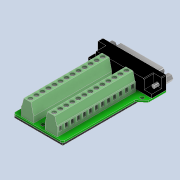
# Autodesk Inventor part: 25Pin D SUB Male Connector
Saved by Autodesk Inventor 2022 (Build 260153000, 153)
## iProperties
Created: 2021-12-24
Part Number: 25Pin D SUB Male Connector
Material: Generic
Document SubType Name: Modeling
Designer: Coy
Density: 1 g/cm^3
Appearance: Anodized - Black
Author: Coy
Autodesk Inventor part; units mm, degrees
ref_plane "YZ Plane" through (0, 0, 0) normal (1, 0, 0) x (0, 1, 0)
ref_plane "XZ Plane" through (0, 0, 0) normal (0, 1, 0) x (-1, 0, 0)
sketch "Sketch1" plane through (0, 0, 0) normal (0, 1, 0) x (-1, 0, 0)
  line L0 (0, 0) -> (53, 0)
  line L1 (53, 0) -> (53, -80)
  line L2 (53, -80) -> (0, -80)
  line L3 (0, -80) -> (0, 0)
  line L4 (47, 0) -> (47, -60)
  line L5 (47, -60) -> (53, -65)
  line L6 (26.5, -80) -> (26.5, 0) construction
  line L7 (6, 0) -> (6, -60)
  line L8 (6, -60) -> (0, -65)
  dimension "d0" = 53
  dimension "d1" = 80
  dimension "d2" = 60
  dimension "d3" = 6
  dimension "d4" = 15
  constraints: 18 end point, 3 symmetric about line, 2 midpoint, 2 parallel, 2 point on line, 1 horizontal, 1 perpendicular, 1 vertical
  measures "d0" distance of L1.end L2.end
  measures "d1" distance of L0.end L1.end
  measures "d2" distance of L4.start L4.end
  measures "d3" distance between parallel lines of L1 L4
  measures "d4" distance of L1.end L5.end
extrude "Extrusion1" add sketch "Sketch1" along normal blind 1.5 contours L0 L4 L5 L1 L2 L3 L8 L7
sketch "Sketch2" plane through (0, 0, 0) normal (0, -1, 0) x (1, 0, 0)
  line L0 (-46.5, -0.5) -> (-6.5, -0.5)
  line L1 (-6.5, -0.5) -> (-6.5, -79.5)
  line L2 (-6.5, -79.5) -> (-46.5, -79.5)
  line L3 (-46.5, -79.5) -> (-46.5, -0.5)
  line L4 (-47, 0) -> (-6, 0) projected
  line L5 (-47, -60) -> (-47, 0) projected
  line L6 (-6, 0) -> (-6, -60) projected
  line L7 (0, -80) -> (-53, -80) projected
  point P0 (0, 0)
  dimension "d7" = 0.5
  dimension "d8" = 0.5
  dimension "d9" = 0.5
  dimension "d10" = 0.5
  constraints: 8 end point, 2 parallel, 1 horizontal, 1 perpendicular
  measures "d7" distance between parallel lines of L4 L0
  measures "d8" distance between parallel lines of L5 L3
  measures "d9" distance between parallel lines of L6 L1
  measures "d10" distance between parallel lines of L7 L2
extrude "Extrusion2" add sketch "Sketch2" along normal blind 2
sketch "Sketch3" plane through (0, 1.5, 0) normal (0, 1, 0) x (1, 0, 0)
  line L0 (-4.625, -3.6868) -> (-4.625, 83.4711) construction
  line L1 (-48.625, -3.6868) -> (-48.625, 83.4711) construction
  line L2 (0, 65) -> (0, 80) construction
  line L3 (15.3473, 64.5) -> (-90.3777, 64.5) construction
  line L4 (0, 80) -> (-53, 80) construction
  line L5 (0, 80) -> (-53, 80) construction
  line L6 (-26.5, 80) -> (-26.5, 0) construction
  line L7 (-47, 0) -> (-6, 0) construction
  line L8 (-6, 0) -> (-6, 60) construction
  line L9 (-6, 4) -> (-47, 4) construction
  line L10 (-47, 60) -> (-47, 0) construction
  circle A0 centre (-26.5, 4) radius 1.625
  circle A1 centre (-4.625, 64.5) radius 1.625
  circle A2 centre (-48.625, 64.5) radius 1.625
  point P0 (0, 0)
  dimension "d13" = 44
  dimension "d14" = 4.625
  dimension "d15" = 15.5
  dimension "d16" = 4
  dimension "d17" = 3.25
  dimension "d18" = 3.25
  dimension "d19" = 3.25
  constraints: 10 end point, 6 point on line, 3 centre point, 3 midpoint, 2 horizontal, 2 vertical
  measures "d13" distance between parallel lines of L1 L0
  measures "d14" distance between parallel lines of L2 L0
  measures "d15" distance between parallel lines of L4 L3
  measures "d16" distance between parallel lines of L7 L9
  measures "d17" diameter of A0
  measures "d18" diameter of A1
  measures "d19" diameter of A2
extrude "Extrusion3" cut sketch "Sketch3" against normal up to surface (1.5 mm away)
sketch "Sketch4" plane through (0, 1.5, 0) normal (0, 1, 0) x (1, 0, 0)
  line L0 (-53, 80) -> (-53, 65) projected
  line L1 (0, 65) -> (0, 80) projected
  line L2 (-53, 80) -> (0, 80)
  line L3 (0, 80) -> (0, 68)
  line L4 (0, 68) -> (-53, 68)
  line L5 (-53, 68) -> (-53, 80)
  point P0 (0, 0)
  dimension "d22" = 12
  constraints: 8 end point, 2 parallel, 1 horizontal, 1 perpendicular, 1 point on line
  measures "d22" distance of L2.end L3.end
extrude "Extrusion4" add sketch "Sketch4" along normal blind 3
sketch "Sketch5" plane through (0, 4.5, 0) normal (0, 1, 0) x (1, 0, 0)
  line L0 (-53, 80) -> (-53, 68) projected
  line L1 (-53, 68) -> (0, 68) projected
  line L2 (0, 68) -> (0, 80) projected
  line L3 (0, 80) -> (-53, 80) projected
  line L4 (-53, 80) -> (-53, 65) projected
  line L5 (-53, 76) -> (0.4812, 76)
  line L6 (-46.5, 76) -> (-46.5, 68)
  line L7 (0, 68) -> (-53, 68) projected
  line L8 (-6.5, 76) -> (-6.5, 68)
  point P0 (0, 0)
  point P1 (0, 76)
  dimension "d25" = 4
  dimension "d26" = 6.5
  dimension "d27" = 6.5
  constraints: 6 end point, 5 point on line, 2 perpendicular, 1 horizontal
  measures "d25" distance between parallel lines of L3 L5
  measures "d26" distance between parallel lines of L0 L6
  measures "d27" distance between parallel lines of L2 L8
extrude "Extrusion5" add sketch "Sketch5" along normal blind 8 contours L3 L2 L5 L0 | L5 L8 L1 L6
sketch "Sketch6" plane through (0, 0, -80) normal (0, 0, -1) x (-1, 0, 0)
  line L0 (7.25, 10.25) -> (45.75, 10.25)
  line L1 (43.75, 2.25) -> (9.25, 2.25)
  line L2 (43.75, 10.25) -> (43.75, 2.25) construction
  line L3 (9.25, 10.25) -> (9.25, 2.25) construction
  line L4 (7.25, 10.25) -> (9.25, 2.25)
  line L5 (43.75, 2.25) -> (45.75, 10.25)
  line L6 (46.5, 12.5) -> (6.5, 12.5) construction
  line L7 (26.5, 12.5) -> (26.5, -2) construction
  line L8 (46.5, -2) -> (6.5, -2) construction
  line L9 (0, 0) -> (0, 12.5) construction
  line L10 (0, 6.25) -> (53, 6.25) construction
  line L11 (53, 0) -> (53, 12.5) construction
  line L12 (4.527, 8.575) -> (5.8694, 6.25)
  line L13 (5.8694, 6.25) -> (4.527, 3.925)
  line L14 (4.527, 3.925) -> (1.8423, 3.925)
  line L15 (1.8423, 3.925) -> (0.5, 6.25)
  line L16 (0.5, 6.25) -> (1.8423, 8.575)
  line L17 (1.8423, 8.575) -> (4.527, 8.575)
  line L18 (51.1577, 8.575) -> (52.5, 6.25)
  line L19 (52.5, 6.25) -> (51.1577, 3.925)
  line L20 (51.1577, 3.925) -> (48.473, 3.925)
  line L21 (48.473, 3.925) -> (47.1306, 6.25)
  line L22 (47.1306, 6.25) -> (48.473, 8.575)
  line L23 (48.473, 8.575) -> (51.1577, 8.575)
  point P0 (3.1847, 6.25)
  point P1 (49.8153, 6.25)
  point P2 (49.8153, 8.575)
  dimension "d34" = 38.5
  dimension "d35" = 8
  dimension "d36" = 104.036
  dimension "d37" = 104.036
  dimension "d38" = 19.25
  dimension "d39" = 4
  dimension "d40" = 4.65
  dimension "d41" = 4.65
  dimension "d42" = 0.5
  dimension "d43" = 0.5
  constraints: 40 end point, 5 midpoint, 5 point on line, 2 horizontal, 2 perpendicular, 1 parallel, 26 other
  measures "d34" distance of L0.start L0.end
  measures "d35" distance between parallel lines of L1 L0
  measures "d36" angle of L1 L4
  measures "d37" angle of L1 L5
  measures "d38" distance from line of L7 L0.end
  measures "d39" distance between parallel lines of L10 L0
  measures "d40" distance between parallel lines of L14 L17
  measures "d41" distance between parallel lines of L20 L23
  measures "d42" distance from line of L11 L18.end
  measures "d43" distance of L10.start L15.end
extrude "Extrusion6" add sketch "Sketch6" along normal blind 6.25
sketch "Sketch7" plane through (0, 0, -86.25) normal (0, 0, -1) x (-1, 0, 0)
  line L0 (1.8423, 8.575) -> (0.5, 6.25) projected
  line L1 (0.5, 6.25) -> (1.8423, 3.925) projected
  line L2 (1.8423, 3.925) -> (4.527, 3.925) projected
  line L3 (4.527, 3.925) -> (5.8694, 6.25) projected
  line L4 (5.8694, 6.25) -> (4.527, 8.575) projected
  line L5 (4.527, 8.575) -> (1.8423, 8.575) projected
  line L6 (48.473, 8.575) -> (47.1306, 6.25) projected
  line L7 (47.1306, 6.25) -> (48.473, 3.925) projected
  line L8 (48.473, 3.925) -> (51.1577, 3.925) projected
  line L9 (51.1577, 3.925) -> (52.5, 6.25) projected
  line L10 (52.5, 6.25) -> (51.1577, 8.575) projected
  line L11 (51.1577, 8.575) -> (48.473, 8.575) projected
  circle A0 centre (3.1847, 6.25) radius 1.25
  circle A1 centre (49.8153, 6.25) radius 1.25
  line L12 (45.75, 10.25) -> (7.25, 10.25) projected
  line L13 (7.25, 10.25) -> (9.25, 2.25) projected
  line L14 (9.25, 2.25) -> (43.75, 2.25) projected
  line L15 (43.75, 2.25) -> (45.75, 10.25) projected
  line L16 (7.8904, 9.75) -> (45.1096, 9.75)
  line L17 (45.1096, 9.75) -> (43.3596, 2.75)
  line L18 (43.3596, 2.75) -> (9.6404, 2.75)
  line L19 (9.6404, 2.75) -> (7.8904, 9.75)
  line L20 (9.6404, 7.25) -> (43.3596, 7.25) construction
  line L21 (9.6404, 5.25) -> (43.3596, 5.25) construction
  circle A2 centre (9.6404, 7.25) radius 0.5
  circle A3 centre (12.4404, 7.25) radius 0.5
  circle A4 centre (15.2404, 7.25) radius 0.5
  circle A5 centre (18.0404, 7.25) radius 0.5
  circle A6 centre (20.8404, 7.25) radius 0.5
  circle A7 centre (23.6404, 7.25) radius 0.5
  circle A8 centre (26.4404, 7.25) radius 0.5
  circle A9 centre (29.2404, 7.25) radius 0.5
  circle A10 centre (32.0404, 7.25) radius 0.5
  circle A11 centre (34.8404, 7.25) radius 0.5
  circle A12 centre (37.6404, 7.25) radius 0.5
  circle A13 centre (40.4404, 7.25) radius 0.5
  circle A14 centre (43.2404, 7.25) radius 0.5
  circle A15 centre (11.0404, 5.25) radius 0.5
  circle A16 centre (13.8404, 5.25) radius 0.5
  circle A17 centre (16.6404, 5.25) radius 0.5
  circle A18 centre (19.4404, 5.25) radius 0.5
  circle A19 centre (22.2404, 5.25) radius 0.5
  circle A20 centre (25.0404, 5.25) radius 0.5
  circle A21 centre (27.8404, 5.25) radius 0.5
  circle A22 centre (30.6404, 5.25) radius 0.5
  circle A23 centre (33.4404, 5.25) radius 0.5
  circle A24 centre (36.2404, 5.25) radius 0.5
  circle A25 centre (39.0404, 5.25) radius 0.5
  circle A26 centre (41.8404, 5.25) radius 0.5
  point P0 (0, 0)
  dimension "d46" = 2.5
  dimension "d47" = 2.5
  dimension "d48" = 0.5
  dimension "d49" = 3
  dimension "d50" = 3
  dimension "d51" = 1
  dimension "d54" = 2.8
  dimension "d59" = 1
  dimension "d60" = 1.4
  dimension "d63" = 2.8
  constraints: 27 centre point, 12 end point, 3 horizontal, 1 coincident, 1 parallel, 1 point on line, 49 other
  measures "d46" diameter of A0
  measures "d47" diameter of A1
  measures "d48" distance between parallel lines of L12 L16
  measures "d49" distance between parallel lines of L12 L20
  measures "d50" distance between parallel lines of L14 L21
  measures "d51" diameter of A2
  measures "d54" distance of A2.centre A3.centre
  measures "d59" diameter of A15
  measures "d60" horizontal distance of L20.start A15.centre
  measures "d63" distance of A15.centre A16.centre
extrude "Extrusion7" cut sketch "Sketch7" against normal up to surface (6.25 mm away) contours A0 | A1 | L16 L17 L18 L19
sketch "Sketch8" plane through (-6.5, 4.5, -76) normal (0, 0, 1) x (1, 0, 0)
  circle A0 centre (-43.3153, 1.75) radius 1.25 projected
  circle A1 centre (3.3153, 1.75) radius 1.25 projected
  circle A2 centre (-43.3153, 1.75) radius 1.25 projected
  circle A3 centre (-43.3153, 1.75) radius 1.5
  circle A4 centre (3.3153, 1.75) radius 1.25 projected
  circle A5 centre (3.3153, 1.75) radius 1.5
  point P0 (6.5, -4.5)
  dimension "d70" = 3
  dimension "d71" = 3
  constraints: 2 centre point, 2 coincident
  measures "d70" diameter of A3
  measures "d71" diameter of A5
extrude "Extrusion8" add sketch "Sketch8" along normal blind 3.5 contours A0 | A1 | A3 | A5
ref_plane "Work Plane1" through (-47, 0, -1) normal (0, 0, 1) x (1, 0, 0)
sketch "Sketch9" plane through (-47, 0, -1) normal (0, 0, 1) x (1, 0, 0)
  line L0 (47, 0) -> (-6, 0) construction
  line L1 (20.5, 0) -> (20.5, 19.9001) construction
  line L2 (47, 1.5) -> (-6, 1.5) construction
  line L3 (5.5, 1.5) -> (5.5, 9.25)
  line L4 (5.5, 9.25) -> (6, 9.25)
  line L5 (6, 9.25) -> (7.625, 15.5)
  line L6 (7.625, 15.5) -> (13.625, 15.5)
  line L7 (13.625, 15.5) -> (15.75, 6.5)
  line L8 (15.75, 6.5) -> (15.75, 1.5)
  line L9 (0, 1.5) -> (41, 1.5) projected
  line L10 (5.5, 2.0746) -> (15.75, 2.0746) construction
  line L11 (10.625, 2.0746) -> (10.625, 15.5) construction
  line L12 (0, 0) -> (0, 1.5) construction
  line L13 (35.5, 1.5) -> (35.5, 9.25)
  line L14 (35.5, 9.25) -> (35, 9.25)
  line L15 (35, 9.25) -> (33.375, 15.5)
  line L16 (33.375, 15.5) -> (27.375, 15.5)
  line L17 (27.375, 15.5) -> (25.25, 6.5)
  line L18 (25.25, 6.5) -> (25.25, 1.5)
  line L19 (35.5, 2.0746) -> (25.25, 2.0746) construction
  line L20 (30.375, 2.0746) -> (30.375, 15.5) construction
  dimension "d75" = 14
  dimension "d76" = 7.75
  dimension "d77" = 0.5
  dimension "d78" = 5
  dimension "d79" = 6
  dimension "d80" = 10.25
  dimension "d81" = 5.5
  constraints: 34 end point, 11 symmetric about line, 6 point on line, 3 midpoint, 3 perpendicular, 2 parallel, 2 vertical
  measures "d75" distance between parallel lines of L2 L6
  measures "d76" distance of L3.start L3.end
  measures "d77" distance of L3.end L4.end
  measures "d78" distance of L7.end L8.end
  measures "d79" distance of L5.end L6.end
  measures "d80" distance of L8.end L3.start
  measures "d81" distance between parallel lines of L12 L3
extrude "Extrusion9" add sketch "Sketch9" against normal blind 65
sketch "Sketch10" plane through (-19.625, 15.5, -1) normal (0, 1, 0) x (1, 0, 0)
  line L0 (-21.875, 65) -> (-11.625, 65) construction
  line L1 (-16.75, 65) -> (-16.75, 0) construction
  line L2 (-11.625, 0) -> (-21.875, 0) construction
  line L3 (-27.375, -1) -> (13.625, -1) construction
  line L4 (-6.3154, 85.25) -> (-7.3154, 85.25) construction
  line L5 (-6.875, -1) -> (-6.875, 85.2511) construction
  circle A0 centre (-16.75, 2.5) radius 1.875
  circle A1 centre (-16.75, 7.5) radius 1.875
  circle A2 centre (-16.75, 12.5) radius 1.875
  circle A3 centre (-16.75, 17.5) radius 1.875
  circle A4 centre (-16.75, 22.5) radius 1.875
  circle A5 centre (-16.75, 27.5) radius 1.875
  circle A6 centre (-16.75, 32.5) radius 1.875
  circle A7 centre (-16.75, 37.5) radius 1.875
  circle A8 centre (-16.75, 42.5) radius 1.875
  circle A9 centre (-16.75, 47.5) radius 1.875
  circle A10 centre (-16.75, 52.5) radius 1.875
  circle A11 centre (-16.75, 57.5) radius 1.875
  circle A12 centre (-16.75, 62.5) radius 1.875
  line L6 (3, 65) -> (3, 0) construction
  circle A13 centre (3, 2.5) radius 1.875
  circle A14 centre (3, 7.5) radius 1.875
  circle A15 centre (3, 12.5) radius 1.875
  circle A16 centre (3, 17.5) radius 1.875
  circle A17 centre (3, 22.5) radius 1.875
  circle A18 centre (3, 27.5) radius 1.875
  circle A19 centre (3, 32.5) radius 1.875
  circle A20 centre (3, 37.5) radius 1.875
  circle A21 centre (3, 42.5) radius 1.875
  circle A22 centre (3, 47.5) radius 1.875
  circle A23 centre (3, 52.5) radius 1.875
  circle A24 centre (3, 57.5) radius 1.875
  circle A25 centre (3, 62.5) radius 1.875
  point P0 (19.625, -1)
  point P1 (-2.125, 65)
  point P2 (-2.125, 0)
  dimension "d84" = 3.75
  dimension "d85" = 2.5
  dimension "d88" = 5
  constraints: 26 centre point, 17 symmetric about line, 6 end point, 3 midpoint, 2 point on line, 1 perpendicular, 1 vertical, 37 other
  measures "d84" diameter of A0
  measures "d85" distance from line of L2 A0.centre
  measures "d88" distance of A0.centre A1.centre
extrude "Extrusion10" cut sketch "Sketch10" against normal blind 1.5
sketch "Sketch11" plane through (-11.5, 1.5, -1) normal (1, 0, 0) x (0, 0, -1)
  line L0 (1.25, 6.75) -> (3.75, 6.75)
  line L1 (3.75, 6.75) -> (3.75, 2.75)
  line L2 (3.75, 2.75) -> (1.25, 2.75)
  line L3 (1.25, 2.75) -> (1.25, 6.75)
  line L4 (0.625, 14) -> (4.375, 14) construction
  line L5 (2.5, 14) -> (2.5, 0) construction
  line L6 (59, 0) -> (-1, 0) construction
  line L7 (0, 7.75) -> (65, 7.75) construction
  line L8 (6.25, 6.75) -> (8.75, 6.75)
  line L9 (8.75, 6.75) -> (8.75, 2.75)
  line L10 (8.75, 2.75) -> (6.25, 2.75)
  line L11 (6.25, 2.75) -> (6.25, 6.75)
  line L12 (7.5, 14) -> (7.5, 0) construction
  line L13 (11.25, 6.75) -> (13.75, 6.75)
  line L14 (13.75, 6.75) -> (13.75, 2.75)
  line L15 (13.75, 2.75) -> (11.25, 2.75)
  line L16 (11.25, 2.75) -> (11.25, 6.75)
  line L17 (12.5, 14) -> (12.5, 0) construction
  line L18 (16.25, 6.75) -> (18.75, 6.75)
  line L19 (18.75, 6.75) -> (18.75, 2.75)
  line L20 (18.75, 2.75) -> (16.25, 2.75)
  line L21 (16.25, 2.75) -> (16.25, 6.75)
  line L22 (17.5, 14) -> (17.5, 0) construction
  line L23 (21.25, 6.75) -> (23.75, 6.75)
  line L24 (23.75, 6.75) -> (23.75, 2.75)
  line L25 (23.75, 2.75) -> (21.25, 2.75)
  line L26 (21.25, 2.75) -> (21.25, 6.75)
  line L27 (22.5, 14) -> (22.5, 0) construction
  line L28 (26.25, 6.75) -> (28.75, 6.75)
  line L29 (28.75, 6.75) -> (28.75, 2.75)
  line L30 (28.75, 2.75) -> (26.25, 2.75)
  line L31 (26.25, 2.75) -> (26.25, 6.75)
  line L32 (27.5, 14) -> (27.5, 0) construction
  line L33 (31.25, 6.75) -> (33.75, 6.75)
  line L34 (33.75, 6.75) -> (33.75, 2.75)
  line L35 (33.75, 2.75) -> (31.25, 2.75)
  line L36 (31.25, 2.75) -> (31.25, 6.75)
  line L37 (32.5, 14) -> (32.5, 0) construction
  line L38 (36.25, 6.75) -> (38.75, 6.75)
  line L39 (38.75, 6.75) -> (38.75, 2.75)
  line L40 (38.75, 2.75) -> (36.25, 2.75)
  line L41 (36.25, 2.75) -> (36.25, 6.75)
  line L42 (37.5, 14) -> (37.5, 0) construction
  line L43 (41.25, 6.75) -> (43.75, 6.75)
  line L44 (43.75, 6.75) -> (43.75, 2.75)
  line L45 (43.75, 2.75) -> (41.25, 2.75)
  line L46 (41.25, 2.75) -> (41.25, 6.75)
  line L47 (42.5, 14) -> (42.5, 0) construction
  line L48 (46.25, 6.75) -> (48.75, 6.75)
  line L49 (48.75, 6.75) -> (48.75, 2.75)
  line L50 (48.75, 2.75) -> (46.25, 2.75)
  line L51 (46.25, 2.75) -> (46.25, 6.75)
  line L52 (47.5, 14) -> (47.5, 0) construction
  line L53 (51.25, 6.75) -> (53.75, 6.75)
  line L54 (53.75, 6.75) -> (53.75, 2.75)
  line L55 (53.75, 2.75) -> (51.25, 2.75)
  line L56 (51.25, 2.75) -> (51.25, 6.75)
  line L57 (52.5, 14) -> (52.5, 0) construction
  line L58 (56.25, 6.75) -> (58.75, 6.75)
  line L59 (58.75, 6.75) -> (58.75, 2.75)
  line L60 (58.75, 2.75) -> (56.25, 2.75)
  line L61 (56.25, 2.75) -> (56.25, 6.75)
  line L62 (57.5, 14) -> (57.5, 0) construction
  line L63 (61.25, 6.75) -> (63.75, 6.75)
  line L64 (63.75, 6.75) -> (63.75, 2.75)
  line L65 (63.75, 2.75) -> (61.25, 2.75)
  line L66 (61.25, 2.75) -> (61.25, 6.75)
  line L67 (62.5, 14) -> (62.5, 0) construction
  point P0 (-1, -1.5)
  dimension "d95" = 2.5
  dimension "d96" = 4
  dimension "d97" = 1.25
  dimension "d98" = 1
  dimension "d101" = 5
  constraints: 130 end point, 2 horizontal, 2 parallel, 1 midpoint, 1 perpendicular, 1 point on line, 1 vertical, 132 other
  measures "d95" distance of L1.end L2.end
  measures "d96" distance of L0.end L1.end
  measures "d97" distance between parallel lines of L5 L1
  measures "d98" distance between parallel lines of L7 L0
  measures "d101" distance of L0.start L8.start
extrude "Extrusion11" cut sketch "Sketch11" against normal blind 2
sketch "Sketch12" plane through (-41.5, 1.5, -1) normal (-1, 0, 0) x (0, 0, 1)
  line L0 (-13.75, 6.75) -> (-13.75, 2.75) projected
  line L1 (-13.75, 2.75) -> (-11.25, 2.75) projected
  line L2 (-11.25, 2.75) -> (-11.25, 6.75) projected
  line L3 (-11.25, 6.75) -> (-13.75, 6.75) projected
  line L4 (-33.75, 6.75) -> (-33.75, 2.75) projected
  line L5 (-33.75, 2.75) -> (-31.25, 2.75) projected
  line L6 (-31.25, 2.75) -> (-31.25, 6.75) projected
  line L7 (-31.25, 6.75) -> (-33.75, 6.75) projected
  line L8 (-53.75, 6.75) -> (-53.75, 2.75) projected
  line L9 (-53.75, 2.75) -> (-51.25, 2.75) projected
  line L10 (-51.25, 2.75) -> (-51.25, 6.75) projected
  line L11 (-51.25, 6.75) -> (-53.75, 6.75) projected
  line L12 (-58.75, 6.75) -> (-58.75, 2.75) projected
  line L13 (-58.75, 2.75) -> (-56.25, 2.75) projected
  line L14 (-56.25, 2.75) -> (-56.25, 6.75) projected
  line L15 (-56.25, 6.75) -> (-58.75, 6.75) projected
  line L16 (-38.75, 6.75) -> (-38.75, 2.75) projected
  line L17 (-38.75, 2.75) -> (-36.25, 2.75) projected
  line L18 (-36.25, 2.75) -> (-36.25, 6.75) projected
  line L19 (-36.25, 6.75) -> (-38.75, 6.75) projected
  line L20 (-18.75, 6.75) -> (-18.75, 2.75) projected
  line L21 (-18.75, 2.75) -> (-16.25, 2.75) projected
  line L22 (-16.25, 2.75) -> (-16.25, 6.75) projected
  line L23 (-16.25, 6.75) -> (-18.75, 6.75) projected
  line L24 (-8.75, 6.75) -> (-8.75, 2.75) projected
  line L25 (-8.75, 2.75) -> (-6.25, 2.75) projected
  line L26 (-6.25, 2.75) -> (-6.25, 6.75) projected
  line L27 (-6.25, 6.75) -> (-8.75, 6.75) projected
  line L28 (-28.75, 6.75) -> (-28.75, 2.75) projected
  line L29 (-28.75, 2.75) -> (-26.25, 2.75) projected
  line L30 (-26.25, 2.75) -> (-26.25, 6.75) projected
  line L31 (-26.25, 6.75) -> (-28.75, 6.75) projected
  line L32 (-48.75, 6.75) -> (-48.75, 2.75) projected
  line L33 (-48.75, 2.75) -> (-46.25, 2.75) projected
  line L34 (-46.25, 2.75) -> (-46.25, 6.75) projected
  line L35 (-46.25, 6.75) -> (-48.75, 6.75) projected
  line L36 (-63.75, 6.75) -> (-63.75, 2.75) projected
  line L37 (-63.75, 2.75) -> (-61.25, 2.75) projected
  line L38 (-61.25, 2.75) -> (-61.25, 6.75) projected
  line L39 (-61.25, 6.75) -> (-63.75, 6.75) projected
  line L40 (-43.75, 6.75) -> (-43.75, 2.75) projected
  line L41 (-43.75, 2.75) -> (-41.25, 2.75) projected
  line L42 (-41.25, 2.75) -> (-41.25, 6.75) projected
  line L43 (-41.25, 6.75) -> (-43.75, 6.75) projected
  line L44 (-23.75, 6.75) -> (-23.75, 2.75) projected
  line L45 (-23.75, 2.75) -> (-21.25, 2.75) projected
  line L46 (-21.25, 2.75) -> (-21.25, 6.75) projected
  line L47 (-21.25, 6.75) -> (-23.75, 6.75) projected
  line L48 (-3.75, 6.75) -> (-3.75, 2.75) projected
  line L49 (-3.75, 2.75) -> (-1.25, 2.75) projected
  line L50 (-1.25, 2.75) -> (-1.25, 6.75) projected
  line L51 (-1.25, 6.75) -> (-3.75, 6.75) projected
  line L52 (0, 0) -> (0, 7.75) projected
  line L53 (-65, 0) -> (0, 0) projected
  line L54 (-65, 7.75) -> (-65, 0) projected
  line L55 (0, 7.75) -> (-65, 7.75) projected
  point P0 (1, -1.5)
extrude "Extrusion12" cut sketch "Sketch12" against normal blind 2 contours L3 L2 L1 L0 | L7 L6 L5 L4 | L11 L10 L9 L8 | L15 L14 L13 L12 | L19 L18 L17 L16 | L23 L22 L21 L20 | L27 L26 L25 L24 | L31 L30 L29 L28 | L35 L34 L33 L32 | L39 L38 L37 L36 | L43 L42 L41 L40 | L47 L46 L45 L44 | L51 L50 L49 L48
fillet "Fillet1" radius 2 8 edges at (-45.1096, 9.75, -83.125) (-43.3596, 2.75, -83.125) (-7.8904, 9.75, -83.125) (-9.6404, 2.75, -83.125) (-7.25, 10.25, -83.125) (-9.25, 2.25, -83.125) (-45.75, 10.25, -83.125) (-43.75, 2.25, -83.125)
fillet "Fillet2" radius 0.5 4 edges at (-6.5, 12.5, -72) (0, 12.5, -78) (-46.5, 12.5, -72) (-53, 12.5, -78)
sketch "Sketch13" plane through (0, 0, -65) normal (1, 0, 0) x (0, 0, -1)
  line L0 (11, 12) -> (15, 12) projected
  line L1 (11, 4.5) -> (11, 12) projected
  line L2 (3, 4.5) -> (11, 4.5) projected
  line L3 (3, 1.5) -> (3, 4.5) projected
  line L4 (0, 1.5) -> (3, 1.5) projected
  line L5 (0, 0) -> (0, 1.5) projected
  line L6 (0, 0) -> (15, 0) projected
  line L7 (15, 0) -> (15, 12) projected
  line L8 (3, 1.5) -> (3, 4.5) projected
  line L9 (3, 1.5) -> (15, 1.5)
  line L10 (15, 0) -> (15, 12) projected
  point P0 (-65, 0)
  constraints: 2 end point, 1 horizontal, 1 point on line
extrude "Extrusion13" cut sketch "Sketch13" against normal blind 0.0001 contours L0 L7 L9 L3 L2 L1
sketch "Sketch14" plane through (0, 0, -80) normal (0, 0, -1) x (-1, 0, 0)
  line L0 (0, 12) -> (0.0001, 12) projected
  line L1 (0.0001, 12) -> (0.0001, 1.5) projected
  line L2 (0.0001, 1.5) -> (0, 1.5) projected
  line L3 (0, 0) -> (0, 1.5) projected
  line L4 (0, 0) -> (53, 0) projected
  line L5 (53, 0) -> (53, 12) projected
  arc A0 (53, 12) -> (52.5, 12.5) centre (52.5, 12) ccw projected
  line L6 (0.5, 12.5) -> (52.5, 12.5) projected
  arc A1 (0.5, 12.5) -> (0, 12) centre (0.5, 12) ccw projected
  line L7 (1.8423, 8.575) -> (4.527, 8.575) projected
  line L8 (4.527, 8.575) -> (5.8694, 6.25) projected
  line L9 (5.8694, 6.25) -> (4.527, 3.925) projected
  line L10 (4.527, 3.925) -> (1.8423, 3.925) projected
  line L11 (1.8423, 3.925) -> (0.5, 6.25) projected
  line L12 (0.5, 6.25) -> (1.8423, 8.575) projected
  line L13 (45.1287, 7.7649) -> (44.1287, 3.7649) projected
  arc A2 (42.1884, 2.25) -> (44.1287, 3.7649) centre (42.1884, 4.25) ccw projected
  line L14 (42.1884, 2.25) -> (10.8116, 2.25) projected
  arc A3 (8.8713, 3.7649) -> (10.8116, 2.25) centre (10.8116, 4.25) ccw projected
  line L15 (8.8713, 3.7649) -> (7.8713, 7.7649) projected
  arc A4 (9.8116, 10.25) -> (7.8713, 7.7649) centre (9.8116, 8.25) ccw projected
  line L16 (9.8116, 10.25) -> (43.1884, 10.25) projected
  arc A5 (45.1287, 7.7649) -> (43.1884, 10.25) centre (43.1884, 8.25) ccw projected
  line L17 (48.473, 8.575) -> (51.1577, 8.575) projected
  line L18 (51.1577, 8.575) -> (52.5, 6.25) projected
  line L19 (52.5, 6.25) -> (51.1577, 3.925) projected
  line L20 (51.1577, 3.925) -> (48.473, 3.925) projected
  line L21 (48.473, 3.925) -> (47.1306, 6.25) projected
  line L22 (47.1306, 6.25) -> (48.473, 8.575) projected
  line L23 (0, 1.5) -> (53, 1.5)
  line L24 (53, 1.5) -> (47, 1.5) projected
  constraints: 2 end point, 1 collinear, 1 point on line
extrude "Extrusion14" cut sketch "Sketch14" against normal blind 0.0001 contours A1 L6 A0 L5 L23 L1
sketch "Sketch15" plane through (-53, 0, -80) normal (-1, 0, 0) x (0, 0, 1)
  line L0 (0.0001, 1.5) -> (0.0001, 12) projected
  line L1 (4, 12) -> (0.0001, 12) projected
  line L2 (4, 4.5) -> (4, 12) projected
  line L3 (12, 4.5) -> (4, 4.5) projected
  line L4 (12, 1.5) -> (12, 4.5) projected
  line L5 (0.0001, 1.5) -> (12, 1.5) projected
  point P0 (80, 0)
extrude "Extrusion15" cut sketch "Sketch15" against normal blind 0.0001
fillet "Fillet3" radius 0.5 25 edges at (-9.1404, 7.25, -86.25) (-11.9404, 7.25, -86.25) (-13.3404, 5.25, -86.25) (-10.5404, 5.25, -86.25) (-14.7404, 7.25, -86.25) (-16.1404, 5.25, -86.25) (-17.5404, 7.25, -86.25) (-18.9404, 5.25, -86.25) (-20.3404, 7.25, -86.25) (-21.7404, 5.25, -86.25) (-23.1404, 7.25, -86.25) (-24.5404, 5.25, -86.25) (-27.3404, 5.25, -86.25) (-25.9404, 7.25, -86.25) (-28.7404, 7.25, -86.25) (-30.1404, 5.25, -86.25) (-31.5404, 7.25, -86.25) (-32.9404, 5.25, -86.25) (-34.3404, 7.25, -86.25) (-35.7404, 5.25, -86.25) (-37.1404, 7.25, -86.25) (-38.5404, 5.25, -86.25) (-39.9404, 7.25, -86.25) (-41.3404, 5.25, -86.25) (-42.7404, 7.25, -86.25)
thread "Thread1" size "M3x0.5" class "6g" standard "ANSI Metric M Profile" full length
thread "Thread2" size "M3x0.5" class "6g" standard "ANSI Metric M Profile" full length
chamfer "Chamfer1" distance 1.5 angle 45 26 edges at (-13.5, 8.25, -63.5) (-13.5, 8.25, -58.5) (-13.5, 8.25, -53.5) (-13.5, 8.25, -48.5) (-13.5, 8.25, -43.5) (-13.5, 8.25, -38.5) (-13.5, 8.25, -33.5) (-13.5, 8.25, -28.5) (-13.5, 8.25, -23.5) (-13.5, 8.25, -18.5) (-13.5, 8.25, -13.5) (-13.5, 8.25, -8.5) (-13.5, 8.25, -3.5) (-39.5, 8.25, -63.5) (-39.5, 8.25, -58.5) (-39.5, 8.25, -53.5) (-39.5, 8.25, -48.5) (-39.5, 8.25, -43.5) (-39.5, 8.25, -38.5) (-39.5, 8.25, -33.5) (-39.5, 8.25, -28.5) (-39.5, 8.25, -23.5) (-39.5, 8.25, -18.5) (-39.5, 8.25, -13.5) (-39.5, 8.25, -8.5) (-39.5, 8.25, -3.5)
fillet "Fillet4" radius 0.5 2 edges at (-11.5, 9.25, -33.5) (-41.5, 9.25, -33.5)
sketch "Sketch16" plane through (-36.375, 14, -3.5) normal (0, 1, 0) x (1, 0, 0)
  circle A0 centre (0, 0) radius 1.875 construction
  line L0 (-1.3258, -1.3258) -> (1.3258, 1.3258) construction
  line L1 (0, 0) -> (0, -4.6267) construction
  line L2 (-1.538, -1.1137) -> (1.1137, 1.538)
  line L3 (-1.1137, -1.538) -> (1.538, 1.1137)
  circle A1 centre (0, 0) radius 1.875
  line L4 (-1.1137, 3.462) -> (1.538, 6.1137)
  line L5 (-1.538, 3.8863) -> (1.1137, 6.538)
  circle A2 centre (0, 5) radius 1.875
  line L6 (-1.1137, 8.462) -> (1.538, 11.1137)
  line L7 (-1.538, 8.8863) -> (1.1137, 11.538)
  circle A3 centre (0, 10) radius 1.875
  line L8 (-1.1137, 13.462) -> (1.538, 16.1137)
  line L9 (-1.538, 13.8863) -> (1.1137, 16.538)
  circle A4 centre (0, 15) radius 1.875
  line L10 (-1.1137, 18.462) -> (1.538, 21.1137)
  line L11 (-1.538, 18.8863) -> (1.1137, 21.538)
  circle A5 centre (0, 20) radius 1.875
  line L12 (-1.1137, 23.462) -> (1.538, 26.1137)
  line L13 (-1.538, 23.8863) -> (1.1137, 26.538)
  circle A6 centre (0, 25) radius 1.875
  line L14 (-1.1137, 28.462) -> (1.538, 31.1137)
  line L15 (-1.538, 28.8863) -> (1.1137, 31.538)
  circle A7 centre (0, 30) radius 1.875
  line L16 (-1.1137, 33.462) -> (1.538, 36.1137)
  line L17 (-1.538, 33.8863) -> (1.1137, 36.538)
  circle A8 centre (0, 35) radius 1.875
  line L18 (-1.1137, 38.462) -> (1.538, 41.1137)
  line L19 (-1.538, 38.8863) -> (1.1137, 41.538)
  circle A9 centre (0, 40) radius 1.875
  line L20 (-1.1137, 43.462) -> (1.538, 46.1137)
  line L21 (-1.538, 43.8863) -> (1.1137, 46.538)
  circle A10 centre (0, 45) radius 1.875
  line L22 (-1.1137, 48.462) -> (1.538, 51.1137)
  line L23 (-1.538, 48.8863) -> (1.1137, 51.538)
  circle A11 centre (0, 50) radius 1.875
  line L24 (-1.1137, 53.462) -> (1.538, 56.1137)
  line L25 (-1.538, 53.8863) -> (1.1137, 56.538)
  circle A12 centre (0, 55) radius 1.875
  line L26 (-1.1137, 58.462) -> (1.538, 61.1137)
  line L27 (-1.538, 58.8863) -> (1.1137, 61.538)
  circle A13 centre (0, 60) radius 1.875
  line L28 (-9.625, 64.5) -> (29.375, 64.5) construction
  line L29 (9.875, 64.5) -> (9.875, -4.875) construction
  circle A14 centre (19.75, 0) radius 1.875 construction
  line L30 (21.0758, -1.3258) -> (18.4242, 1.3258) construction
  line L31 (21.288, -1.1137) -> (18.6363, 1.538)
  line L32 (20.8637, -1.538) -> (18.212, 1.1137)
  circle A15 centre (19.75, 0) radius 1.875
  line L33 (20.8637, 3.462) -> (18.212, 6.1137)
  line L34 (21.288, 3.8863) -> (18.6363, 6.538)
  circle A16 centre (19.75, 5) radius 1.875
  line L35 (20.8637, 8.462) -> (18.212, 11.1137)
  line L36 (21.288, 8.8863) -> (18.6363, 11.538)
  circle A17 centre (19.75, 10) radius 1.875
  line L37 (20.8637, 13.462) -> (18.212, 16.1137)
  line L38 (21.288, 13.8863) -> (18.6363, 16.538)
  circle A18 centre (19.75, 15) radius 1.875
  line L39 (20.8637, 18.462) -> (18.212, 21.1137)
  line L40 (21.288, 18.8863) -> (18.6363, 21.538)
  circle A19 centre (19.75, 20) radius 1.875
  line L41 (20.8637, 23.462) -> (18.212, 26.1137)
  line L42 (21.288, 23.8863) -> (18.6363, 26.538)
  circle A20 centre (19.75, 25) radius 1.875
  line L43 (20.8637, 28.462) -> (18.212, 31.1137)
  line L44 (21.288, 28.8863) -> (18.6363, 31.538)
  circle A21 centre (19.75, 30) radius 1.875
  line L45 (20.8637, 33.462) -> (18.212, 36.1137)
  line L46 (21.288, 33.8863) -> (18.6363, 36.538)
  circle A22 centre (19.75, 35) radius 1.875
  line L47 (20.8637, 38.462) -> (18.212, 41.1137)
  line L48 (21.288, 38.8863) -> (18.6363, 41.538)
  circle A23 centre (19.75, 40) radius 1.875
  line L49 (20.8637, 43.462) -> (18.212, 46.1137)
  line L50 (21.288, 43.8863) -> (18.6363, 46.538)
  circle A24 centre (19.75, 45) radius 1.875
  line L51 (20.8637, 48.462) -> (18.212, 51.1137)
  line L52 (21.288, 48.8863) -> (18.6363, 51.538)
  circle A25 centre (19.75, 50) radius 1.875
  line L53 (20.8637, 53.462) -> (18.212, 56.1137)
  line L54 (21.288, 53.8863) -> (18.6363, 56.538)
  circle A26 centre (19.75, 55) radius 1.875
  line L55 (20.8637, 58.462) -> (18.212, 61.1137)
  line L56 (21.288, 58.8863) -> (18.6363, 61.538)
  circle A27 centre (19.75, 60) radius 1.875
  point P0 (36.375, -3.5)
  point P1 (18.6534, 1.5209)
  point P2 (18.2291, 1.0966)
  point P3 (20.8466, -1.5209)
  point P4 (21.2709, -1.0966)
  point P5 (18.6534, 6.5209)
  point P6 (18.2291, 6.0966)
  point P7 (20.8466, 3.4791)
  point P8 (21.2709, 3.9034)
  point P9 (18.6534, 11.5209)
  point P10 (18.2291, 11.0966)
  point P11 (20.8466, 8.4791)
  point P12 (21.2709, 8.9034)
  point P13 (18.6534, 16.5209)
  point P14 (18.2291, 16.0966)
  point P15 (20.8466, 13.4791)
  point P16 (21.2709, 13.9034)
  point P17 (18.6534, 21.5209)
  point P18 (18.2291, 21.0966)
  point P19 (20.8466, 18.4791)
  point P20 (21.2709, 18.9034)
  point P21 (18.6534, 26.5209)
  point P22 (18.2291, 26.0966)
  point P23 (20.8466, 23.4791)
  point P24 (21.2709, 23.9034)
  point P25 (18.6534, 31.5209)
  point P26 (18.2291, 31.0966)
  point P27 (20.8466, 28.4791)
  point P28 (21.2709, 28.9034)
  point P29 (21.2709, 33.9034)
  point P30 (18.6534, 36.5209)
  point P31 (18.2291, 36.0966)
  point P32 (20.8466, 33.4791)
  point P33 (18.6534, 41.5209)
  point P34 (18.2291, 41.0966)
  point P35 (20.8466, 38.4791)
  point P36 (21.2709, 38.9034)
  point P37 (18.2291, 46.0966)
  point P38 (20.8466, 43.4791)
  point P39 (21.2709, 43.9034)
  point P40 (18.6534, 46.5209)
  point P41 (18.6534, 51.5209)
  point P42 (18.2291, 51.0966)
  point P43 (20.8466, 48.4791)
  point P44 (21.2709, 48.9034)
  point P45 (18.6534, 56.5209)
  point P46 (18.2291, 56.0966)
  point P47 (20.8466, 53.4791)
  point P48 (21.2709, 53.9034)
  point P49 (21.2709, 58.9034)
  point P50 (18.6534, 61.5209)
  point P51 (18.2291, 61.0966)
  point P52 (20.8466, 58.4791)
  point P53 (1.5209, 61.0966)
  point P54 (1.0966, 61.5209)
  point P55 (-1.5209, 58.9034)
  point P56 (-1.0966, 58.4791)
  point P57 (1.5209, 56.0966)
  point P58 (1.0966, 56.5209)
  point P59 (-1.5209, 53.9034)
  point P60 (-1.0966, 53.4791)
  point P61 (1.5209, 51.0966)
  point P62 (1.0966, 51.5209)
  point P63 (-1.5209, 48.9034)
  point P64 (-1.0966, 48.4791)
  point P65 (1.5209, 46.0966)
  point P66 (1.0966, 46.5209)
  point P67 (-1.5209, 43.9034)
  point P68 (-1.0966, 43.4791)
  point P69 (1.5209, 41.0966)
  point P70 (1.0966, 41.5209)
  point P71 (-1.5209, 38.9034)
  point P72 (-1.0966, 38.4791)
  point P73 (1.5209, 36.0966)
  point P74 (1.0966, 36.5209)
  point P75 (-1.5209, 33.9034)
  point P76 (-1.0966, 33.4791)
  point P77 (1.5209, 31.0966)
  point P78 (1.0966, 31.5209)
  point P79 (-1.5209, 28.9034)
  point P80 (-1.0966, 28.4791)
  point P81 (1.5209, 26.0966)
  point P82 (1.0966, 26.5209)
  point P83 (-1.5209, 23.9034)
  point P84 (-1.0966, 23.4791)
  point P85 (1.5209, 21.0966)
  point P86 (1.0966, 21.5209)
  point P87 (-1.5209, 18.9034)
  point P88 (-1.0966, 18.4791)
  point P89 (1.5209, 16.0966)
  point P90 (1.0966, 16.5209)
  point P91 (-1.5209, 13.9034)
  point P92 (-1.0966, 13.4791)
  point P93 (1.5209, 11.0966)
  point P94 (1.0966, 11.5209)
  point P95 (-1.5209, 8.9034)
  point P96 (-1.0966, 8.4791)
  point P97 (1.5209, 6.0966)
  point P98 (1.0966, 6.5209)
  point P99 (-1.5209, 3.9034)
  point P100 (-1.0966, 3.4791)
  point P101 (1.5209, 1.0966)
  point P102 (1.0966, 1.5209)
  point P103 (-1.5209, -1.0966)
  point P104 (-1.0966, -1.5209)
  dimension "d127" = 45
  dimension "d128" = 0.3
  dimension "d129" = 0.3
  dimension "d132" = 5
  constraints: 112 end point, 68 symmetric about line, 27 centre point, 4 point on circle, 3 midpoint, 3 vertical, 2 coincident, 2 parallel, 1 concentric, 110 other
  measures "d127" angle of L1 L0
  measures "d128" distance between parallel lines of L0 L2
  measures "d129" distance between parallel lines of L0 L3
  measures "d132" distance of L3.start L4.start
extrude "Extrusion16" cut sketch "Sketch16" against normal blind 0.5 contours L2 A1 L3 | A2 L5 L4 | A3 L7 L6 | A4 L9 L8 | A5 L11 L10 | A6 L13 L12 | A7 L15 L14 | A8 L17 L16 | A9 L19 L18 | A10 L21 L20 | A11 L23 L22 | A12 L25 L24 | A13 L27 L26 | A15 L32 L31 | L33 A16 L34 | L35 A17 L36 | L37 A18 L38 | L39 A19 L40 | L41 A20 L42 | L43 A21 L44 | L45 A22 L46 | L47 A23 L48 | L49 A24 L50 | L51 A25 L52 | L53 A26 L54 | L55 A27 L56
fillet "Fillet5" radius 1.6 2 edges at (-6, 0.75, 0) (-47, 0.75, 0)
equation "\"d8\" = d7"
equation "\"d9\" = d7"
equation "\"d10\" = d7"
equation "\"d18\" = d17"
equation "\"d19\" = d17"
equation "\"d27\" = d26"
equation "\"d38\" = 0.5 * d34"
equation "\"d39\" = 0.5 * d35"
equation "\"d41\" = d40"
equation "\"d43\" = d42"
equation "\"d47\" = d46"
equation "\"d50\" = d49"
equation "\"d59\" = d51"
equation "\"d60\" = 0.5 * d54"
equation "\"d71\" = d70"
equation "\"d97\" = 0.5 * d95"
body "Solid1"
